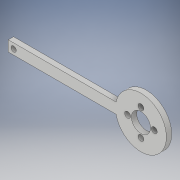
# Autodesk Inventor part: ClawLinkage
Saved by Autodesk Inventor 2017 (Build 210142000, 142)
## iProperties
Created: 2017-09-29
Part Number: ClawLinkage
Material: Generic
Document SubType Name: Modeling
Designer: User
Density: 1 g/cm^3
Appearance: Default
Author: User
Autodesk Inventor part; units mm, degrees
ref_plane "YZ Plane" through (0, 0, 0) normal (1, 0, 0) x (0, 1, 0)
ref_plane "XZ Plane" through (0, 0, 0) normal (0, 1, 0) x (-1, 0, 0)
ref_plane "XY Plane" through (0, 0, 0) normal (0, 0, 1) x (1, 0, 0)
sketch "Sketch1" plane through (0, 0, 0) normal (0, 0, 1) x (1, 0, 0)
  circle A0 centre (0, 0) radius 15.24
  line L0 (0, 0) -> (-8.001, 0)
  line L1 (0, 0) -> (8.001, 0)
  line L2 (0, 0) -> (0, 8.001)
  line L3 (0, 0) -> (0, -8.001)
  circle A1 centre (8.001, 0) radius 1.7526
  circle A2 centre (0, 8.001) radius 1.7526
  circle A3 centre (-8.001, 0) radius 1.7526
  circle A4 centre (0, -8.001) radius 1.7526
  dimension "d0" = 30.48
  dimension "d11" = 8.001
  dimension "d12" = 8.001
  dimension "d13" = 8.001
  dimension "d14" = 8.001
  dimension "d15" = 3.5052
  dimension "d16" = 3.5052
  dimension "d17" = 3.5052
  dimension "d18" = 3.5052
  constraints: 8 end point, 5 centre point, 5 coincident, 2 horizontal, 2 vertical
  measures "d0" diameter of A0
  measures "d11" distance of L0.start L0.end
  measures "d12" distance of L0.start L1.end
  measures "d13" distance of L0.start L2.end
  measures "d14" distance of L0.start L3.end
  measures "d15" diameter of A1
  measures "d16" diameter of A2
  measures "d17" diameter of A3
  measures "d18" diameter of A4
extrude "Extrusion1" add sketch "Sketch1" along normal blind 3.175 contours A0 | A1 | A2 | A3 | A4
sketch "Sketch2" plane through (0, 0, 3.175) normal (0, 0, 1) x (1, 0, 0)
  circle A0 centre (0, 0) radius 15.24 projected
  line L0 (-15.24, 0) -> (-15.24, 3.175)
  line L1 (-15.24, 0) -> (-15.24, -3.175)
  dimension "d3" = 3.175
  dimension "d4" = 3.175
  constraints: 4 end point, 4 vertical, 1 horizontal alignment, 1 other
  measures "d3" distance of L0.start L0.end
  measures "d4" distance of L0.start L1.end
ref_plane "Work Plane1" through (-15.24, 0, 3.175) normal (1, 0, 0) x (0, 1, 0)
sketch "Sketch3" plane through (-15.24, 0, 3.175) normal (1, 0, 0) x (0, 1, 0)
  line L0 (15.24, 0) -> (-15.24, 0) projected
  line L1 (-15.24, -3.175) -> (15.24, -3.175) projected
  line L2 (0, -3.175) -> (3.175, -3.175)
  line L3 (3.175, -3.175) -> (3.175, 0)
  line L4 (3.175, 0) -> (-3.175, 0)
  line L5 (-3.175, 0) -> (-3.175, -3.175)
  line L6 (-3.175, -3.175) -> (3.175, -3.175)
  dimension "d6" = 6.35
  constraints: 10 end point, 3 perpendicular, 1 collinear, 1 point on line
  measures "d6" distance of L3.end L4.end
extrude "Extrusion2" add sketch "Sketch3" against normal blind 64.2493
sketch "Sketch4" plane through (-15.24, 0, 3.175) normal (1, 0, 0) x (0, 0, -1)
  line L0 (3.175, -3.175) -> (3.175, 0) projected
  line L1 (0, 3.175) -> (3.175, 3.175)
  line L2 (3.175, 3.175) -> (3.175, -3.175)
  line L3 (3.175, -3.175) -> (0, -3.175)
  line L4 (0, -3.175) -> (0, 3.175)
  constraints: 8 end point, 2 parallel, 1 horizontal, 1 perpendicular
extrude "Extrusion3" add sketch "Sketch4" along normal blind 12.7
extrude "Extrusion4" cut sketch "Sketch1" along normal blind 12.7 contours A1 | A2 | A3 | A4
sketch "Sketch5" plane through (0, 0, 0) normal (0, 0, -1) x (-1, 0, 0)
  circle A0 centre (0, 0) radius 5.715
  dimension "d21" = 11.43
  constraints: 1 centre point, 1 coincident
  measures "d21" diameter of A0
extrude "Extrusion5" cut sketch "Sketch5" against normal blind 12.7
sketch "Sketch7" plane through (0, 0, 3.175) normal (0, 0, 1) x (1, 0, 0)
  line L0 (-79.4893, -3.175) -> (-79.4893, 3.175) projected
  line L1 (-79.4893, 0) -> (-76.3143, 0)
  circle A0 centre (-76.3143, 0) radius 1.5875
  point P0 (0, 0)
  dimension "d26" = 3.175
  dimension "d27" = 3.175
  constraints: 2 end point, 1 centre point, 1 coincident, 1 horizontal, 1 midpoint
  measures "d26" distance of L1.start L1.end
  measures "d27" diameter of A0
extrude "Extrusion7" cut sketch "Sketch7" against normal blind 3.175
body "Solid1"
